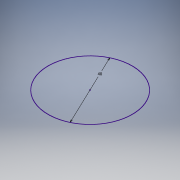
# Autodesk Inventor part: フランジ
Saved by Autodesk Inventor 2019 (Build 230136000, 136)
## iProperties
Created: 2020-10-25
Part Number: フランジ
Material: 一般
Document SubType Name: Modeling
Designer: zhept
Density: 1 g/cm^3
Appearance: 既定
Author: zhept
Autodesk Inventor part; units mm, degrees
ref_plane "YZ Plane" through (0, 0, 0) normal (1, 0, 0) x (0, 1, 0)
ref_plane "XZ Plane" through (0, 0, 0) normal (0, 1, 0) x (-1, 0, 0)
ref_plane "XY Plane" through (0, 0, 0) normal (0, 0, 1) x (1, 0, 0)
sketch "スケッチ1" plane through (0, 0, 0) normal (0, 1, 0) x (-1, 0, 0)
  circle A0 centre (0, 0) radius 17.5
  line L0 (0, 0) -> (0, 8)
  line L1 (0, 0) -> (-8, 0)
  line L2 (0, 0) -> (0, -8)
  circle A1 centre (0, -8) radius 2.15
  circle A2 centre (0, 8) radius 2.15
  circle A3 centre (-8, 0) radius 2.15
  dimension "d0" = 35
  dimension "d1" = 8
  dimension "d2" = 8
  dimension "d4" = 8
  dimension "d5" = 4.3
  dimension "d6" = 4.3
  dimension "d7" = 4.3
  constraints: 6 end point, 4 centre point, 4 coincident, 2 vertical, 1 horizontal
  measures "d0" diameter of A0
  measures "d1" distance of L0.start L0.end
  measures "d2" distance of L0.start L1.end
  measures "d4" distance of L0.start L2.end
  measures "d5" diameter of A1
  measures "d6" diameter of A2
  measures "d7" diameter of A3
extrude "押し出し1" add sketch "スケッチ1" along normal blind 3
